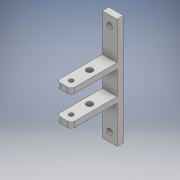
# Autodesk Inventor part: Część1
Saved by Autodesk Inventor 2017 (Build 210142000, 142)
## iProperties
Created: 2019-10-19
Part Number: Część1
Material: Ogólny
Document SubType Name: Modeling
Designer: patry
Density: 1 g/cm^3
Appearance: Domyślna
Author: patry
Autodesk Inventor part; units mm, degrees
ref_plane "YZ Plane" through (0, 0, 0) normal (1, 0, 0) x (0, 1, 0)
ref_plane "XZ Plane" through (0, 0, 0) normal (0, 1, 0) x (-1, 0, 0)
ref_plane "XY Plane" through (0, 0, 0) normal (0, 0, 1) x (1, 0, 0)
sketch "Szkic1" plane through (0, 0, 0) normal (0, 1, 0) x (-1, 0, 0)
  line L0 (-4, 30) -> (4, 30)
  line L1 (4, 30) -> (4, -30)
  line L2 (4, -30) -> (-4, -30)
  line L3 (-4, -30) -> (-4, 30)
  line L4 (-4, 30) -> (4, -30) construction
  line L5 (4, 30) -> (-4, -30) construction
  circle A0 centre (0, 25) radius 1.5
  circle A1 centre (0, -25) radius 1.5
  point P0 (0, 0)
  dimension "d0" = 8
  dimension "d1" = 60
  dimension "d2" = 50
  dimension "d3" = 5
  dimension "d4" = 4
  dimension "d5" = 3
  dimension "d6" = 3
  constraints: 12 end point, 2 centre point, 2 coincident, 2 midpoint, 2 parallel, 1 horizontal, 1 perpendicular, 1 vertical alignment
  measures "d0" distance of L1.end L2.end
  measures "d1" distance of L0.end L1.end
  measures "d2" distance of point (0, -25) point (0, 25)
  measures "d3" distance from line of L0 point (0, 25)
  measures "d4" distance from line of L1 point (0, 25)
  measures "d5" diameter of A0
  measures "d6" diameter of A1
extrude "Wyciągnięcie proste1" add sketch "Szkic1" along normal blind 3.5
sketch "Szkic2" plane through (0, 0, 0) normal (0, -1, 0) x (1, 0, 0)
  line L0 (4, 30) -> (4, -30) projected
  line L1 (-4, -9.5) -> (4, -9.5)
  line L2 (4, -9.5) -> (4, -6.5)
  line L3 (4, -6.5) -> (-4, -6.5)
  line L4 (-4, -6.5) -> (-4, -9.5)
  line L5 (-4, 6.5) -> (4, 6.5)
  line L6 (4, 6.5) -> (4, 9.5)
  line L7 (4, 9.5) -> (-4, 9.5)
  line L8 (-4, 9.5) -> (-4, 6.5)
  point P0 (0, 0)
  dimension "d9" = 3
  dimension "d10" = 3
  dimension "d11" = 13
  dimension "d12" = 6.5
  constraints: 16 end point, 4 parallel, 2 horizontal, 2 perpendicular, 2 point on line
  measures "d9" distance between parallel lines of L3 L1
  measures "d10" distance between parallel lines of L7 L5
  measures "d11" distance between parallel lines of L5 L3
  measures "d12" distance from line of point (0, 0) L3
extrude "Wyciągnięcie proste2" add sketch "Szkic2" along normal blind 25
fillet "Zaokrąglenie1" radius 2 4 edges at (4, -25, -8) (-4, -25, -8) (4, -25, 8) (-4, -25, 8)
sketch "Szkic3" plane through (-4, 0, 9.5) normal (0, 0, 1) x (1, 0, 0)
  line L0 (0, 0) -> (0, -23) projected
  line L1 (6, -25) -> (2, -25) projected
  point P0 (4, 0)
  point P1 (4, -21)
  point P2 (4, -11)
  dimension "d16" = 10
  dimension "d17" = 4
  dimension "d18" = 4
  measures "d16" distance of point (4, -21) point (4, -11)
  measures "d17" distance from line of L0 point (4, -21)
  measures "d18" distance from line of L1 point (4, -21)
hole "Otwór1" at (0, -11, 9.5) direction (0, 0, -1) diameter 3.4 end through all clearance for "Śruba ze łbem płaskim obrobiona" size "M3" standard "ANSI Profil metryczny M"
hole "Otwór2" at (0, -21, 9.5) direction (0, 0, -1) diameter 2.4 end through all clearance for "Śruba ze łbem płaskim obrobiona" size "M2" standard "ANSI Profil metryczny M"
equation "\"d10\" = d9"
equation "\"d12\" = 0.5 * d11"
